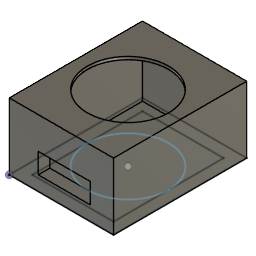
flipdot-joystick (Autodesk Fusion 360 design; units mm, degrees)
Autodesk Fusion 360 part; units mm, degrees
sketch "Sketch1" plane through (0, 0, 0) normal (0, 0, 1) x (1, 0, 0)
  line L0 (4, 4) -> (32, 4)
  line L1 (32, 4) -> (32, 42)
  line L2 (32, 42) -> (4, 42)
  line L3 (4, 42) -> (4, 4)
  line L4 (0, 0) -> (36, 0)
  line L5 (36, 0) -> (36, 46)
  line L6 (36, 46) -> (0, 46)
  line L7 (0, 46) -> (0, 0)
  circle A0 centre (18, 23) radius 14
  dimension "d1" = 28
  dimension "d2" = 38
  dimension "d3" = 36
  dimension "d4" = 46
  dimension "d5" = 4
  dimension "d6" = 4
  constraint horizontal L0
  constraint vertical L1
  constraint horizontal L2
  constraint vertical L3
  constraint horizontal L4
  constraint vertical L5
  constraint horizontal L6
  constraint vertical L7
  constraint coincident L4.start L7.end
  measures "d1" distance of L0.start L0.end
  measures "d2" distance of L0.start L2.end
  measures "d3" distance of L4.start L4.end
  measures "d4" distance of L4.start L6.end
  measures "d5" distance of L2 L6
  measures "d6" distance of L1 L5
extrude "Extrude1" add sketch "Sketch1" along normal blind 23
extrude "Extrude2" add sketch "Sketch1" along normal blind 3 contours L0 L1 L3 A0 | L1 L2 L3 A0 | A0
extrude "Extrude3" add sketch "Sketch1" along normal blind 1 from surface at 22 contours L0 L1 L3 A0 | L1 L2 L3 A0
sketch "Sketch2" plane through (0, 0, 0) normal (0, -1, 0) x (1, 0, 0)
  line L0 (0, 0) -> (36, 0)
  line L1 (36, 0) -> (36, 23)
  line L2 (36, 23) -> (0, 23)
  line L3 (0, 23) -> (0, 0)
  line L4 (10, 12) -> (28, 12)
  line L5 (28, 12) -> (28, 5)
  line L6 (28, 5) -> (10, 5)
  line L7 (10, 5) -> (10, 12)
  line L8 (0, 0) -> (36, 0)
  dimension "d14" = 18
  dimension "d15" = 7
  dimension "d16" = 5
  constraint horizontal L4
  constraint vertical L5
  constraint horizontal L6
  constraint vertical L7
  measures "d14" distance of L4.start L4.end
  measures "d15" distance of L4.start L6.end
  measures "d16" distance of L6 L8
extrude "Extrude4" cut sketch "Sketch2" against normal blind 4 contours L4 L5 L6 L7
